Autodesk Inventor part; units mm, degrees
(part 2 of 2)
  line L376 (6.1518, -23.1931) -> (8.2731, -25.3144) projected
  line L377 (8.2731, -25.3144) -> (6.1518, -27.4357) projected
  line L378 (6.1518, -27.4357) -> (4.0305, -25.3144) projected
  line L379 (4.0305, -25.3144) -> (6.1518, -23.1931) projected
  line L380 (3.7123, -25.6326) -> (5.8336, -27.7539) projected
  line L381 (5.8336, -27.7539) -> (3.7123, -29.8753) projected
  line L382 (3.7123, -29.8753) -> (1.591, -27.7539) projected
  line L383 (1.591, -27.7539) -> (3.7123, -25.6326) projected
  line L384 (1.2728, -28.0721) -> (3.3941, -30.1935) projected
  line L385 (3.3941, -30.1935) -> (1.2728, -32.3148) projected
  line L386 (1.2728, -32.3148) -> (-0.8485, -30.1935) projected
  line L387 (-0.8485, -30.1935) -> (1.2728, -28.0721) projected
  line L388 (-1.1667, -30.5117) -> (0.9546, -32.633) projected
  line L389 (0.9546, -32.633) -> (-1.1667, -34.7543) projected
  line L390 (-1.1667, -34.7543) -> (-3.288, -32.633) projected
  line L391 (-3.288, -32.633) -> (-1.1667, -30.5117) projected
  line L392 (-3.6062, -32.9512) -> (-1.4849, -35.0725) projected
  line L393 (-1.4849, -35.0725) -> (-3.6062, -37.1938) projected
  line L394 (-3.6062, -37.1938) -> (-5.7276, -35.0725) projected
  line L395 (-5.7276, -35.0725) -> (-3.6062, -32.9512) projected
  line L396 (-6.0458, -35.3907) -> (-3.9244, -37.512) projected
  line L397 (-3.9244, -37.512) -> (-6.0458, -39.6333) projected
  line L398 (-6.0458, -39.6333) -> (-8.1671, -37.512) projected
  line L399 (-8.1671, -37.512) -> (-6.0458, -35.3907) projected
  line L400 (-8.4853, -37.8302) -> (-6.364, -39.9515) projected
  line L401 (-6.364, -39.9515) -> (-8.4853, -42.0729) projected
  line L402 (-8.4853, -42.0729) -> (-10.6066, -39.9515) projected
  line L403 (-10.6066, -39.9515) -> (-8.4853, -37.8302) projected
  line L404 (28.1075, -6.1165) -> (30.2288, -8.2378) projected
  line L405 (30.2288, -8.2378) -> (28.1075, -10.3591) projected
  line L406 (28.1075, -10.3591) -> (25.9862, -8.2378) projected
  line L407 (25.9862, -8.2378) -> (28.1075, -6.1165) projected
  line L408 (25.668, -8.556) -> (27.7893, -10.6773) projected
  line L409 (27.7893, -10.6773) -> (25.668, -12.7986) projected
  line L410 (25.668, -12.7986) -> (23.5467, -10.6773) projected
  line L411 (23.5467, -10.6773) -> (25.668, -8.556) projected
  line L412 (23.2285, -10.9955) -> (25.3498, -13.1168) projected
  line L413 (25.3498, -13.1168) -> (23.2285, -15.2382) projected
  line L414 (23.2285, -15.2382) -> (21.1071, -13.1168) projected
  line L415 (21.1071, -13.1168) -> (23.2285, -10.9955) projected
  line L416 (20.7889, -13.435) -> (22.9103, -15.5563) projected
  line L417 (22.9103, -15.5563) -> (20.7889, -17.6777) projected
  line L418 (20.7889, -17.6777) -> (18.6676, -15.5563) projected
  line L419 (18.6676, -15.5563) -> (20.7889, -13.435) projected
  line L420 (18.3494, -15.8745) -> (20.4707, -17.9959) projected
  line L421 (20.4707, -17.9959) -> (18.3494, -20.1172) projected
  line L422 (18.3494, -20.1172) -> (16.2281, -17.9959) projected
  line L423 (16.2281, -17.9959) -> (18.3494, -15.8745) projected
  line L424 (15.9099, -18.3141) -> (18.0312, -20.4354) projected
  line L425 (18.0312, -20.4354) -> (15.9099, -22.5567) projected
  line L426 (15.9099, -22.5567) -> (13.7886, -20.4354) projected
  line L427 (13.7886, -20.4354) -> (15.9099, -18.3141) projected
  line L428 (13.4704, -20.7536) -> (15.5917, -22.8749) projected
  line L429 (15.5917, -22.8749) -> (13.4704, -24.9962) projected
  line L430 (13.4704, -24.9962) -> (11.3491, -22.8749) projected
  line L431 (11.3491, -22.8749) -> (13.4704, -20.7536) projected
  line L432 (11.0309, -23.1931) -> (13.1522, -25.3144) projected
  line L433 (13.1522, -25.3144) -> (11.0309, -27.4357) projected
  line L434 (11.0309, -27.4357) -> (8.9095, -25.3144) projected
  line L435 (8.9095, -25.3144) -> (11.0309, -23.1931) projected
  line L436 (8.5913, -25.6326) -> (10.7127, -27.7539) projected
  line L437 (10.7127, -27.7539) -> (8.5913, -29.8753) projected
  line L438 (8.5913, -29.8753) -> (6.47, -27.7539) projected
  line L439 (6.47, -27.7539) -> (8.5913, -25.6326) projected
  line L440 (6.1518, -28.0721) -> (8.2731, -30.1935) projected
  line L441 (8.2731, -30.1935) -> (6.1518, -32.3148) projected
  line L442 (6.1518, -32.3148) -> (4.0305, -30.1935) projected
  line L443 (4.0305, -30.1935) -> (6.1518, -28.0721) projected
  line L444 (3.7123, -30.5117) -> (5.8336, -32.633) projected
  line L445 (5.8336, -32.633) -> (3.7123, -34.7543) projected
  line L446 (3.7123, -34.7543) -> (1.591, -32.633) projected
  line L447 (1.591, -32.633) -> (3.7123, -30.5117) projected
  line L448 (1.2728, -32.9512) -> (3.3941, -35.0725) projected
  line L449 (3.3941, -35.0725) -> (1.2728, -37.1938) projected
  line L450 (1.2728, -37.1938) -> (-0.8485, -35.0725) projected
  line L451 (-0.8485, -35.0725) -> (1.2728, -32.9512) projected
  line L452 (-1.1667, -35.3907) -> (0.9546, -37.512) projected
  line L453 (0.9546, -37.512) -> (-1.1667, -39.6333) projected
  line L454 (-1.1667, -39.6333) -> (-3.288, -37.512) projected
  line L455 (-3.288, -37.512) -> (-1.1667, -35.3907) projected
  line L456 (-3.6062, -37.8302) -> (-1.4849, -39.9515) projected
  line L457 (-1.4849, -39.9515) -> (-3.6062, -42.0729) projected
  line L458 (-3.6062, -42.0729) -> (-5.7276, -39.9515) projected
  line L459 (-5.7276, -39.9515) -> (-3.6062, -37.8302) projected
  line L460 (30.547, -8.556) -> (32.6683, -10.6773) projected
  line L461 (32.6683, -10.6773) -> (30.547, -12.7986) projected
  line L462 (30.547, -12.7986) -> (28.4257, -10.6773) projected
  line L463 (28.4257, -10.6773) -> (30.547, -8.556) projected
  line L464 (28.1075, -10.9955) -> (30.2288, -13.1168) projected
  line L465 (30.2288, -13.1168) -> (28.1075, -15.2382) projected
  line L466 (28.1075, -15.2382) -> (25.9862, -13.1168) projected
  line L467 (25.9862, -13.1168) -> (28.1075, -10.9955) projected
  line L468 (25.668, -13.435) -> (27.7893, -15.5563) projected
  line L469 (27.7893, -15.5563) -> (25.668, -17.6777) projected
  line L470 (25.668, -17.6777) -> (23.5467, -15.5563) projected
  line L471 (23.5467, -15.5563) -> (25.668, -13.435) projected
  line L472 (23.2285, -15.8745) -> (25.3498, -17.9959) projected
  line L473 (25.3498, -17.9959) -> (23.2285, -20.1172) projected
  line L474 (23.2285, -20.1172) -> (21.1071, -17.9959) projected
  line L475 (21.1071, -17.9959) -> (23.2285, -15.8745) projected
  line L476 (15.9099, -23.1931) -> (18.0312, -25.3144) projected
  line L477 (18.0312, -25.3144) -> (15.9099, -27.4357) projected
  line L478 (15.9099, -27.4357) -> (13.7886, -25.3144) projected
  line L479 (13.7886, -25.3144) -> (15.9099, -23.1931) projected
  line L480 (13.4704, -25.6326) -> (15.5917, -27.7539) projected
  line L481 (15.5917, -27.7539) -> (13.4704, -29.8753) projected
  line L482 (13.4704, -29.8753) -> (11.3491, -27.7539) projected
  line L483 (11.3491, -27.7539) -> (13.4704, -25.6326) projected
  line L484 (11.0309, -28.0721) -> (13.1522, -30.1935) projected
  line L485 (13.1522, -30.1935) -> (11.0309, -32.3148) projected
  line L486 (11.0309, -32.3148) -> (8.9095, -30.1935) projected
  line L487 (8.9095, -30.1935) -> (11.0309, -28.0721) projected
  line L488 (8.5913, -30.5117) -> (10.7127, -32.633) projected
  line L489 (10.7127, -32.633) -> (8.5913, -34.7543) projected
  line L490 (8.5913, -34.7543) -> (6.47, -32.633) projected
  line L491 (6.47, -32.633) -> (8.5913, -30.5117) projected
  line L492 (6.1518, -32.9512) -> (8.2731, -35.0725) projected
  line L493 (8.2731, -35.0725) -> (6.1518, -37.1938) projected
  line L494 (6.1518, -37.1938) -> (4.0305, -35.0725) projected
  line L495 (4.0305, -35.0725) -> (6.1518, -32.9512) projected
  line L496 (3.7123, -35.3907) -> (5.8336, -37.512) projected
  line L497 (5.8336, -37.512) -> (3.7123, -39.6333) projected
  line L498 (3.7123, -39.6333) -> (1.591, -37.512) projected
  line L499 (1.591, -37.512) -> (3.7123, -35.3907) projected
  line L500 (1.2728, -37.8302) -> (3.3941, -39.9515) projected
  line L501 (3.3941, -39.9515) -> (1.2728, -42.0729) projected
  line L502 (1.2728, -42.0729) -> (-0.8485, -39.9515) projected
  line L503 (-0.8485, -39.9515) -> (1.2728, -37.8302) projected
  line L504 (32.9865, -10.9955) -> (35.1079, -13.1168) projected
  line L505 (35.1079, -13.1168) -> (32.9865, -15.2382) projected
  line L506 (32.9865, -15.2382) -> (30.8652, -13.1168) projected
  line L507 (30.8652, -13.1168) -> (32.9865, -10.9955) projected
  line L508 (13.4704, -30.5117) -> (15.5917, -32.633) projected
  line L509 (15.5917, -32.633) -> (13.4704, -34.7543) projected
  line L510 (13.4704, -34.7543) -> (11.3491, -32.633) projected
  line L511 (11.3491, -32.633) -> (13.4704, -30.5117) projected
  line L512 (11.0309, -32.9512) -> (13.1522, -35.0725) projected
  line L513 (13.1522, -35.0725) -> (11.0309, -37.1938) projected
  line L514 (11.0309, -37.1938) -> (8.9095, -35.0725) projected
  line L515 (8.9095, -35.0725) -> (11.0309, -32.9512) projected
  line L516 (8.5913, -35.3907) -> (10.7127, -37.512) projected
  line L517 (10.7127, -37.512) -> (8.5913, -39.6333) projected
  line L518 (8.5913, -39.6333) -> (6.47, -37.512) projected
  line L519 (6.47, -37.512) -> (8.5913, -35.3907) projected
  line L520 (6.1518, -37.8302) -> (8.2731, -39.9515) projected
  line L521 (8.2731, -39.9515) -> (6.1518, -42.0729) projected
  line L522 (6.1518, -42.0729) -> (4.0305, -39.9515) projected
  line L523 (4.0305, -39.9515) -> (6.1518, -37.8302) projected
  line L524 (35.426, -13.435) -> (37.5474, -15.5563) projected
  line L525 (37.5474, -15.5563) -> (35.426, -17.6777) projected
  line L526 (35.426, -17.6777) -> (33.3047, -15.5563) projected
  line L527 (33.3047, -15.5563) -> (35.426, -13.435) projected
  line L528 (28.1075, -20.7536) -> (30.2288, -22.8749) projected
  line L529 (30.2288, -22.8749) -> (28.1075, -24.9962) projected
  line L530 (28.1075, -24.9962) -> (25.9862, -22.8749) projected
  line L531 (25.9862, -22.8749) -> (28.1075, -20.7536) projected
  line L532 (25.668, -23.1931) -> (27.7893, -25.3144) projected
  line L533 (27.7893, -25.3144) -> (25.668, -27.4357) projected
  line L534 (25.668, -27.4357) -> (23.5467, -25.3144) projected
  line L535 (23.5467, -25.3144) -> (25.668, -23.1931) projected
  line L536 (23.2285, -25.6326) -> (25.3498, -27.7539) projected
  line L537 (25.3498, -27.7539) -> (23.2285, -29.8753) projected
  line L538 (23.2285, -29.8753) -> (21.1071, -27.7539) projected
  line L539 (21.1071, -27.7539) -> (23.2285, -25.6326) projected
  line L540 (18.3494, -30.5117) -> (20.4707, -32.633) projected
  line L541 (20.4707, -32.633) -> (18.3494, -34.7543) projected
  line L542 (18.3494, -34.7543) -> (16.2281, -32.633) projected
  line L543 (16.2281, -32.633) -> (18.3494, -30.5117) projected
  line L544 (15.9099, -32.9512) -> (18.0312, -35.0725) projected
  line L545 (18.0312, -35.0725) -> (15.9099, -37.1938) projected
  line L546 (15.9099, -37.1938) -> (13.7886, -35.0725) projected
  line L547 (13.7886, -35.0725) -> (15.9099, -32.9512) projected
  line L548 (13.4704, -35.3907) -> (15.5917, -37.512) projected
  line L549 (15.5917, -37.512) -> (13.4704, -39.6333) projected
  line L550 (13.4704, -39.6333) -> (11.3491, -37.512) projected
  line L551 (11.3491, -37.512) -> (13.4704, -35.3907) projected
  line L552 (11.0309, -37.8302) -> (13.1522, -39.9515) projected
  line L553 (13.1522, -39.9515) -> (11.0309, -42.0729) projected
  line L554 (11.0309, -42.0729) -> (8.9095, -39.9515) projected
  line L555 (8.9095, -39.9515) -> (11.0309, -37.8302) projected
  line L556 (8.5913, -40.2697) -> (10.7127, -42.3911) projected
  line L557 (10.7127, -42.3911) -> (8.5913, -44.5124) projected
  line L558 (8.5913, -44.5124) -> (6.47, -42.3911) projected
  line L559 (6.47, -42.3911) -> (8.5913, -40.2697) projected
  line L560 (32.9865, -20.7536) -> (35.1079, -22.8749) projected
  line L561 (35.1079, -22.8749) -> (32.9865, -24.9962) projected
  line L562 (32.9865, -24.9962) -> (30.8652, -22.8749) projected
  line L563 (30.8652, -22.8749) -> (32.9865, -20.7536) projected
  line L564 (30.547, -23.1931) -> (32.6683, -25.3144) projected
  line L565 (32.6683, -25.3144) -> (30.547, -27.4357) projected
  line L566 (30.547, -27.4357) -> (28.4257, -25.3144) projected
  line L567 (28.4257, -25.3144) -> (30.547, -23.1931) projected
  line L568 (28.1075, -25.6326) -> (30.2288, -27.7539) projected
  line L569 (30.2288, -27.7539) -> (28.1075, -29.8753) projected
  line L570 (28.1075, -29.8753) -> (25.9862, -27.7539) projected
  line L571 (25.9862, -27.7539) -> (28.1075, -25.6326) projected
  line L572 (25.668, -28.0721) -> (27.7893, -30.1935) projected
  line L573 (27.7893, -30.1935) -> (25.668, -32.3148) projected
  line L574 (25.668, -32.3148) -> (23.5467, -30.1935) projected
  line L575 (23.5467, -30.1935) -> (25.668, -28.0721) projected
  line L576 (23.2285, -30.5117) -> (25.3498, -32.633) projected
  line L577 (25.3498, -32.633) -> (23.2285, -34.7543) projected
  line L578 (23.2285, -34.7543) -> (21.1071, -32.633) projected
  line L579 (21.1071, -32.633) -> (23.2285, -30.5117) projected
  line L580 (20.7889, -32.9512) -> (22.9103, -35.0725) projected
  line L581 (22.9103, -35.0725) -> (20.7889, -37.1938) projected
  line L582 (20.7889, -37.1938) -> (18.6676, -35.0725) projected
  line L583 (18.6676, -35.0725) -> (20.7889, -32.9512) projected
  line L584 (18.3494, -35.3907) -> (20.4707, -37.512) projected
  line L585 (20.4707, -37.512) -> (18.3494, -39.6333) projected
  line L586 (18.3494, -39.6333) -> (16.2281, -37.512) projected
  line L587 (16.2281, -37.512) -> (18.3494, -35.3907) projected
  line L588 (15.9099, -37.8302) -> (18.0312, -39.9515) projected
  line L589 (18.0312, -39.9515) -> (15.9099, -42.0729) projected
  line L590 (15.9099, -42.0729) -> (13.7886, -39.9515) projected
  line L591 (13.7886, -39.9515) -> (15.9099, -37.8302) projected
  line L592 (13.4704, -40.2697) -> (15.5917, -42.3911) projected
  line L593 (15.5917, -42.3911) -> (13.4704, -44.5124) projected
  line L594 (13.4704, -44.5124) -> (11.3491, -42.3911) projected
  line L595 (11.3491, -42.3911) -> (13.4704, -40.2697) projected
  line L596 (37.8656, -20.7536) -> (39.9869, -22.8749) projected
  line L597 (39.9869, -22.8749) -> (37.8656, -24.9962) projected
  line L598 (37.8656, -24.9962) -> (35.7442, -22.8749) projected
  line L599 (35.7442, -22.8749) -> (37.8656, -20.7536) projected
  line L600 (35.426, -23.1931) -> (37.5474, -25.3144) projected
  line L601 (37.5474, -25.3144) -> (35.426, -27.4357) projected
  line L602 (35.426, -27.4357) -> (33.3047, -25.3144) projected
  line L603 (33.3047, -25.3144) -> (35.426, -23.1931) projected
  line L604 (32.9865, -25.6326) -> (35.1079, -27.7539) projected
  line L605 (35.1079, -27.7539) -> (32.9865, -29.8753) projected
  line L606 (32.9865, -29.8753) -> (30.8652, -27.7539) projected
  line L607 (30.8652, -27.7539) -> (32.9865, -25.6326) projected
  line L608 (30.547, -28.0721) -> (32.6683, -30.1935) projected
  line L609 (32.6683, -30.1935) -> (30.547, -32.3148) projected
  line L610 (30.547, -32.3148) -> (28.4257, -30.1935) projected
  line L611 (28.4257, -30.1935) -> (30.547, -28.0721) projected
  line L612 (28.1075, -30.5117) -> (30.2288, -32.633) projected
  line L613 (30.2288, -32.633) -> (28.1075, -34.7543) projected
  line L614 (28.1075, -34.7543) -> (25.9862, -32.633) projected
  line L615 (25.9862, -32.633) -> (28.1075, -30.5117) projected
  line L616 (25.668, -32.9512) -> (27.7893, -35.0725) projected
  line L617 (27.7893, -35.0725) -> (25.668, -37.1938) projected
  line L618 (25.668, -37.1938) -> (23.5467, -35.0725) projected
  line L619 (23.5467, -35.0725) -> (25.668, -32.9512) projected
  line L620 (23.2285, -35.3907) -> (25.3498, -37.512) projected
  line L621 (25.3498, -37.512) -> (23.2285, -39.6333) projected
  line L622 (23.2285, -39.6333) -> (21.1071, -37.512) projected
  line L623 (21.1071, -37.512) -> (23.2285, -35.3907) projected
  line L624 (18.3494, -40.2697) -> (20.4707, -42.3911) projected
  line L625 (20.4707, -42.3911) -> (18.3494, -44.5124) projected
  line L626 (18.3494, -44.5124) -> (16.2281, -42.3911) projected
  line L627 (16.2281, -42.3911) -> (18.3494, -40.2697) projected
  line L628 (37.8656, -25.6326) -> (39.9869, -27.7539) projected
  line L629 (39.9869, -27.7539) -> (37.8656, -29.8753) projected
  line L630 (37.8656, -29.8753) -> (35.7442, -27.7539) projected
  line L631 (35.7442, -27.7539) -> (37.8656, -25.6326) projected
  line L632 (35.426, -28.0721) -> (37.5474, -30.1935) projected
  line L633 (37.5474, -30.1935) -> (35.426, -32.3148) projected
  line L634 (35.426, -32.3148) -> (33.3047, -30.1935) projected
  line L635 (33.3047, -30.1935) -> (35.426, -28.0721) projected
  line L636 (32.9865, -30.5117) -> (35.1079, -32.633) projected
  line L637 (35.1079, -32.633) -> (32.9865, -34.7543) projected
  line L638 (32.9865, -34.7543) -> (30.8652, -32.633) projected
  line L639 (30.8652, -32.633) -> (32.9865, -30.5117) projected
  line L640 (30.547, -32.9512) -> (32.6683, -35.0725) projected
  line L641 (32.6683, -35.0725) -> (30.547, -37.1938) projected
  line L642 (30.547, -37.1938) -> (28.4257, -35.0725) projected
  line L643 (28.4257, -35.0725) -> (30.547, -32.9512) projected
  line L644 (28.1075, -35.3907) -> (30.2288, -37.512) projected
  line L645 (30.2288, -37.512) -> (28.1075, -39.6333) projected
  line L646 (28.1075, -39.6333) -> (25.9862, -37.512) projected
  line L647 (25.9862, -37.512) -> (28.1075, -35.3907) projected
  line L648 (25.668, -37.8302) -> (27.7893, -39.9515) projected
  line L649 (27.7893, -39.9515) -> (25.668, -42.0729) projected
  line L650 (25.668, -42.0729) -> (23.5467, -39.9515) projected
  line L651 (23.5467, -39.9515) -> (25.668, -37.8302) projected
  line L652 (40.3051, -28.0721) -> (42.4264, -30.1935) projected
  line L653 (42.4264, -30.1935) -> (40.3051, -32.3148) projected
  line L654 (40.3051, -32.3148) -> (38.1838, -30.1935) projected
  line L655 (38.1838, -30.1935) -> (40.3051, -28.0721) projected
  line L656 (37.8656, -30.5117) -> (39.9869, -32.633) projected
  line L657 (39.9869, -32.633) -> (37.8656, -34.7543) projected
  line L658 (37.8656, -34.7543) -> (35.7442, -32.633) projected
  line L659 (35.7442, -32.633) -> (37.8656, -30.5117) projected
  line L660 (35.426, -32.9512) -> (37.5474, -35.0725) projected
  line L661 (37.5474, -35.0725) -> (35.426, -37.1938) projected
  line L662 (35.426, -37.1938) -> (33.3047, -35.0725) projected
  line L663 (33.3047, -35.0725) -> (35.426, -32.9512) projected
  line L664 (32.9865, -35.3907) -> (35.1079, -37.512) projected
  line L665 (35.1079, -37.512) -> (32.9865, -39.6333) projected
  line L666 (32.9865, -39.6333) -> (30.8652, -37.512) projected
  line L667 (30.8652, -37.512) -> (32.9865, -35.3907) projected
  line L668 (30.547, -37.8302) -> (32.6683, -39.9515) projected
  line L669 (32.6683, -39.9515) -> (30.547, -42.0729) projected
  line L670 (30.547, -42.0729) -> (28.4257, -39.9515) projected
  line L671 (28.4257, -39.9515) -> (30.547, -37.8302) projected
  line L672 (40.3051, -32.9512) -> (42.4264, -35.0725) projected
  line L673 (42.4264, -35.0725) -> (40.3051, -37.1938) projected
  line L674 (40.3051, -37.1938) -> (38.1838, -35.0725) projected
  line L675 (38.1838, -35.0725) -> (40.3051, -32.9512) projected
  line L676 (37.8656, -35.3907) -> (39.9869, -37.512) projected
  line L677 (39.9869, -37.512) -> (37.8656, -39.6333) projected
  line L678 (37.8656, -39.6333) -> (35.7442, -37.512) projected
  line L679 (35.7442, -37.512) -> (37.8656, -35.3907) projected
  line L680 (35.426, -37.8302) -> (37.5474, -39.9515) projected
  line L681 (37.5474, -39.9515) -> (35.426, -42.0729) projected
  line L682 (35.426, -42.0729) -> (33.3047, -39.9515) projected
  line L683 (33.3047, -39.9515) -> (35.426, -37.8302) projected
  line L684 (29.4532, -43.8031) -> (30.547, -42.7092) projected
  line L685 (30.547, -42.7092) -> (31.7996, -43.9618) projected
  arc A0 (31.7996, -43.9618) -> (32.4051, -43.9309) centre (31.4663, -31.4663) ccw projected
  line L686 (32.4051, -43.9309) -> (30.8652, -42.3911) projected
  line L687 (30.8652, -42.3911) -> (32.9865, -40.2697) projected
  line L688 (32.9865, -40.2697) -> (35.1079, -42.3911) projected
  line L689 (35.1079, -42.3911) -> (33.7415, -43.7574) projected
  arc A1 (33.7415, -43.7574) -> (43.7574, -33.7415) centre (31.4663, -31.4663) ccw projected
  line L690 (43.7574, -33.7415) -> (42.7446, -34.7543) projected
  line L691 (42.7446, -34.7543) -> (40.6233, -32.633) projected
  line L692 (40.6233, -32.633) -> (42.7446, -30.5117) projected
  line L693 (42.7446, -30.5117) -> (43.9635, -31.7305) projected
  arc A2 (43.9635, -31.7305) -> (43.9606, -31.0913) centre (31.4663, -31.4663) ccw projected
  line L694 (43.9606, -31.0913) -> (43.0628, -30.1935) projected
  line L695 (43.0628, -30.1935) -> (43.8031, -29.4532) projected
  arc A3 (43.8031, -29.4532) -> (43.7034, -28.9164) centre (31.4663, -31.4663) ccw projected
  line L696 (43.7034, -28.9164) -> (42.7446, -29.8753) projected
  line L697 (42.7446, -29.8753) -> (40.6233, -27.7539) projected
  line L698 (40.6233, -27.7539) -> (42.5978, -25.7795) projected
  arc A4 (42.5978, -25.7795) -> (42.376, -25.3648) centre (31.4663, -31.4663) ccw projected
  line L699 (42.376, -25.3648) -> (40.3051, -27.4357) projected
  line L700 (40.3051, -27.4357) -> (38.1838, -25.3144) projected
  line L701 (38.1838, -25.3144) -> (40.3051, -23.1931) projected
  line L702 (40.3051, -23.1931) -> (42.2404, -25.1284) projected
  arc A5 (42.2404, -25.1284) -> (37.4767, -20.5061) centre (31.4663, -31.4663) ccw projected
  line L703 (37.4767, -20.5061) -> (35.426, -22.5567) projected
  line L704 (35.426, -22.5567) -> (33.3047, -20.4354) projected
  line L705 (33.3047, -20.4354) -> (34.4199, -19.3202) projected
  arc A6 (34.4199, -19.3202) -> (33.8985, -19.2052) centre (31.4663, -31.4663) ccw projected
  line L706 (33.8985, -19.2052) -> (32.9865, -20.1172) projected
  line L707 (32.9865, -20.1172) -> (31.8412, -18.9719) projected
  arc A7 (31.8412, -18.9719) -> (31.202, -18.969) centre (31.4663, -31.4663) ccw projected
  line L708 (31.202, -18.969) -> (32.6683, -20.4354) projected
  line L709 (32.6683, -20.4354) -> (30.547, -22.5567) projected
  line L710 (30.547, -22.5567) -> (28.4257, -20.4354) projected
  line L711 (28.4257, -20.4354) -> (29.7807, -19.0804) projected
  arc A8 (29.7807, -19.0804) -> (29.0159, -19.2088) centre (31.4663, -31.4663) ccw projected
  line L712 (29.0159, -19.2088) -> (28.1075, -20.1172) projected
  line L713 (28.1075, -20.1172) -> (27.577, -19.5867) projected
  arc A9 (27.577, -19.5867) -> (27.1055, -19.7516) centre (31.4663, -31.4663) ccw projected
  line L714 (27.1055, -19.7516) -> (27.7893, -20.4354) projected
  line L715 (27.7893, -20.4354) -> (25.668, -22.5567) projected
  line L716 (25.668, -22.5567) -> (24.321, -21.2098) projected
  arc A10 (24.321, -21.2098) -> (23.9519, -21.477) centre (31.4663, -31.4663) ccw projected
  line L717 (23.9519, -21.477) -> (25.3498, -22.8749) projected
  line L718 (25.3498, -22.8749) -> (23.2285, -24.9962) projected
  line L719 (23.2285, -24.9962) -> (21.7878, -23.5556) projected
  arc A11 (21.7878, -23.5556) -> (21.5075, -23.9116) centre (31.4663, -31.4663) ccw projected
  line L720 (21.5075, -23.9116) -> (22.9103, -25.3144) projected
  line L721 (22.9103, -25.3144) -> (20.7889, -27.4357) projected
  line L722 (20.7889, -27.4357) -> (19.9526, -26.5994) projected
  arc A12 (19.9526, -26.5994) -> (19.7708, -27.054) centre (31.4663, -31.4663) ccw projected
  line L723 (19.7708, -27.054) -> (20.4707, -27.7539) projected
  line L724 (20.4707, -27.7539) -> (19.2088, -29.0159) projected
  arc A13 (19.2088, -29.0159) -> (19.0804, -29.7807) centre (31.4663, -31.4663) ccw projected
  line L725 (19.0804, -29.7807) -> (20.7889, -28.0721) projected
  line L726 (20.7889, -28.0721) -> (22.9103, -30.1935) projected
  line L727 (22.9103, -30.1935) -> (20.7889, -32.3148) projected
  line L728 (20.7889, -32.3148) -> (18.6676, -30.1935) projected
  line L729 (18.6676, -30.1935) -> (18.914, -29.9471) projected
  line L730 (18.0124, -30.2123) -> (18.914, -29.9471) projected
  line L731 (18.0124, -30.2123) -> (15.9099, -32.3148) projected
  line L732 (15.9099, -32.3148) -> (13.7886, -30.1935) projected
  line L733 (13.7886, -30.1935) -> (15.9099, -28.0721) projected
  line L734 (15.9099, -28.0721) -> (17.5736, -29.7358) projected
  arc A14 (17.6542, -29.18) -> (17.5736, -29.7358) centre (31.4663, -31.4663) ccw projected
  line L735 (17.6542, -29.18) -> (16.2281, -27.7539) projected
  line L736 (16.2281, -27.7539) -> (18.3494, -25.6326) projected
  line L737 (18.3494, -25.6326) -> (18.6193, -25.9025) projected
  arc A15 (18.8179, -25.4647) -> (18.6193, -25.9025) centre (31.4663, -31.4663) ccw projected
  line L738 (18.8179, -25.4647) -> (18.6676, -25.3144) projected
  line L739 (18.6676, -25.3144) -> (19.124, -24.8581) projected
  arc A16 (20.2276, -23.1181) -> (19.124, -24.8581) centre (31.4663, -31.4663) ccw projected
  line L740 (20.2276, -23.1181) -> (18.3494, -24.9962) projected
  line L741 (18.3494, -24.9962) -> (16.2281, -22.8749) projected
  line L742 (16.2281, -22.8749) -> (18.3494, -20.7536) projected
  line L743 (18.3494, -20.7536) -> (20.4379, -22.8421) projected
  arc A17 (20.7224, -22.4902) -> (20.4379, -22.8421) centre (31.4663, -31.4663) ccw projected
  line L744 (20.7224, -22.4902) -> (18.6676, -20.4354) projected
  line L745 (18.6676, -20.4354) -> (20.7889, -18.3141) projected
  line L746 (20.7889, -18.3141) -> (22.8818, -20.407) projected
  arc A18 (24.8581, -19.124) -> (22.8818, -20.407) centre (31.4663, -31.4663) ccw projected
  line L747 (24.8581, -19.124) -> (25.668, -18.3141) projected
  line L748 (25.668, -18.3141) -> (25.9519, -18.598) projected
  arc A19 (26.4039, -18.4136) -> (25.9519, -18.598) centre (31.4663, -31.4663) ccw projected
  line L749 (26.4039, -18.4136) -> (25.9862, -17.9959) projected
  line L750 (25.9862, -17.9959) -> (28.1075, -15.8745) projected
  line L751 (28.1075, -15.8745) -> (29.7988, -17.5659) projected
  arc A20 (30.378, -17.5086) -> (29.7988, -17.5659) centre (31.4663, -31.4663) ccw projected
  line L752 (30.378, -17.5086) -> (28.4257, -15.5563) projected
  line L753 (28.4257, -15.5563) -> (30.547, -13.435) projected
  line L754 (30.547, -13.435) -> (32.6683, -15.5563) projected
  line L755 (32.6683, -15.5563) -> (30.7396, -17.4851) projected
  arc A21 (31.3946, -17.4664) -> (30.7396, -17.4851) centre (31.4663, -31.4663) ccw projected
  line L756 (31.3946, -17.4664) -> (32.9865, -15.8745) projected
  line L757 (32.9865, -15.8745) -> (35.0428, -17.9308) projected
  arc A22 (35.9531, -18.2047) -> (35.0428, -17.9308) centre (31.4663, -31.4663) ccw projected
  line L758 (35.9531, -18.2047) -> (35.7442, -17.9959) projected
  line L759 (35.7442, -17.9959) -> (37.8656, -15.8745) projected
  line L760 (37.8656, -15.8745) -> (39.248, -17.257) projected
  line L761 (39.248, -17.257) -> (38.2823, -15.6549) projected
  line L762 (38.2823, -15.6549) -> (38.1838, -15.5563) projected
  line L763 (38.1838, -15.5563) -> (38.2082, -15.5319) projected
  line L764 (38.2082, -15.5319) -> (37.9689, -15.1349) projected
  line L765 (37.9689, -15.1349) -> (37.8656, -15.2382) projected
  line L766 (37.8656, -15.2382) -> (35.7442, -13.1168) projected
  line L767 (35.7442, -13.1168) -> (36.3733, -12.4878) projected
  line L768 (36.3733, -12.4878) -> (36.1339, -12.0907) projected
  line L769 (36.1339, -12.0907) -> (35.426, -12.7986) projected
  line L770 (35.426, -12.7986) -> (33.3047, -10.6773) projected
  line L771 (33.3047, -10.6773) -> (34.5384, -9.4437) projected
  line L772 (34.5384, -9.4437) -> (34.299, -9.0466) projected
  line L773 (34.299, -9.0466) -> (32.9865, -10.3591) projected
  line L774 (32.9865, -10.3591) -> (30.8652, -8.2378) projected
  line L775 (30.8652, -8.2378) -> (32.7035, -6.3995) projected
  line L776 (32.7035, -6.3995) -> (32.4641, -6.0025) projected
  line L777 (32.4641, -6.0025) -> (30.547, -7.9196) projected
  line L778 (30.547, -7.9196) -> (28.4257, -5.7983) projected
  line L779 (28.4257, -5.7983) -> (30.547, -3.677) projected
  line L780 (30.547, -3.677) -> (31.8444, -4.9744) projected
  line L781 (31.8444, -4.9744) -> (29.6985, -1.4142) projected
  line L782 (29.6985, -1.4142) -> (15.9099, 12.3744) projected
  line L783 (15.9099, 12.3744) -> (-26.5165, -30.052) projected
  line L784 (-26.5165, -30.052) -> (-12.7279, -43.8406) projected
  line L785 (-12.7279, -43.8406) -> (-11.5531, -43.8841) projected
  line L786 (-11.5531, -43.8841) -> (-13.0461, -42.3911) projected
  line L787 (-13.0461, -42.3911) -> (-10.9248, -40.2697) projected
  line L788 (-10.9248, -40.2697) -> (-8.8035, -42.3911) projected
  line L789 (-8.8035, -42.3911) -> (-10.3414, -43.9289) projected
  line L790 (-10.3414, -43.9289) -> (-9.7277, -43.9516) projected
  line L791 (-9.7277, -43.9516) -> (-8.4853, -42.7092) projected
  line L792 (-8.4853, -42.7092) -> (-7.1474, -44.0471) projected
  line L793 (-7.1474, -44.0471) -> (-6.4866, -44.0716) projected
  line L794 (-6.4866, -44.0716) -> (-8.1671, -42.3911) projected
  line L795 (-8.1671, -42.3911) -> (-6.0458, -40.2697) projected
  line L796 (-6.0458, -40.2697) -> (-3.9244, -42.3911) projected
  line L797 (-3.9244, -42.3911) -> (-5.6364, -44.103) projected
  line L798 (-5.6364, -44.103) -> (-5.0227, -44.1257) projected
  line L799 (-5.0227, -44.1257) -> (-3.6062, -42.7092) projected
  line L800 (-3.6062, -42.7092) -> (-2.0809, -44.2346) projected
  line L801 (-2.0809, -44.2346) -> (-1.4201, -44.259) projected
  line L802 (-1.4201, -44.259) -> (-3.288, -42.3911) projected
  line L803 (-3.288, -42.3911) -> (-1.1667, -40.2697) projected
  line L804 (-1.1667, -40.2697) -> (0.9546, -42.3911) projected
  line L805 (0.9546, -42.3911) -> (-0.9315, -44.2771) projected
  line L806 (-0.9315, -44.2771) -> (-0.3178, -44.2998) projected
  line L807 (-0.3178, -44.2998) -> (1.2728, -42.7092) projected
  line L808 (1.2728, -42.7092) -> (2.9856, -44.422) projected
  line L809 (2.9856, -44.422) -> (3.6464, -44.4465) projected
  line L810 (3.6464, -44.4465) -> (1.591, -42.3911) projected
  line L811 (1.591, -42.3911) -> (3.7123, -40.2697) projected
  line L812 (3.7123, -40.2697) -> (5.8336, -42.3911) projected
  line L813 (5.8336, -42.3911) -> (3.7735, -44.4512) projected
  line L814 (3.7735, -44.4512) -> (4.3872, -44.4739) projected
  line L815 (4.3872, -44.4739) -> (6.1518, -42.7092) projected
  line L816 (6.1518, -42.7092) -> (8.0521, -44.6095) projected
  line L817 (8.0521, -44.6095) -> (9.0921, -44.648) projected
  line L818 (9.0921, -44.648) -> (11.0309, -42.7092) projected
  line L819 (11.0309, -42.7092) -> (13.1186, -44.797) projected
  line L820 (13.1186, -44.797) -> (13.7971, -44.8221) projected
  line L821 (13.7971, -44.8221) -> (15.9099, -42.7092) projected
  line L822 (15.9099, -42.7092) -> (18.0312, -44.8306) projected
  line L823 (18.0312, -44.8306) -> (17.8884, -44.9734) projected
  line L824 (17.8884, -44.9734) -> (18.8459, -45.0089) projected
  line L825 (18.8459, -45.0089) -> (18.6676, -44.8306) projected
  line L826 (18.6676, -44.8306) -> (20.7889, -42.7092) projected
  line L827 (20.7889, -42.7092) -> (22.9103, -44.8306) projected
  line L828 (22.9103, -44.8306) -> (22.5933, -45.1475) projected
  line L829 (22.5933, -45.1475) -> (23.207, -45.1702) projected
  line L830 (23.207, -45.1702) -> (23.2285, -45.1488) projected
  line L831 (23.2285, -45.1488) -> (23.2516, -45.1719) projected
  line L832 (23.2516, -45.1719) -> (23.9124, -45.1963) projected
  line L833 (23.9124, -45.1963) -> (23.5467, -44.8306) projected
  line L834 (23.5467, -44.8306) -> (24.6708, -43.7064) projected
  arc A23 (24.2673, -43.4735) -> (24.6708, -43.7064) centre (31.4663, -31.4663) ccw projected
  line L835 (24.2673, -43.4735) -> (23.2285, -44.5124) projected
  line L836 (23.2285, -44.5124) -> (21.1071, -42.3911) projected
  line L837 (21.1071, -42.3911) -> (21.8536, -41.6445) projected
  arc A24 (21.5315, -41.3303) -> (21.8536, -41.6445) centre (31.4663, -31.4663) ccw projected
  line L838 (21.5315, -41.3303) -> (20.7889, -42.0729) projected
  line L839 (20.7889, -42.0729) -> (18.6676, -39.9515) projected
  line L840 (18.6676, -39.9515) -> (20.7889, -37.8302) projected
  line L841 (20.7889, -37.8302) -> (22.9103, -39.9515) projected
  line L842 (22.9103, -39.9515) -> (22.5921, -40.2697) projected
  arc A25 (22.5921, -40.2697) -> (22.9148, -40.5834) centre (31.4663, -31.4663) ccw projected
  line L843 (22.9148, -40.5834) -> (23.2285, -40.2697) projected
  line L844 (23.2285, -40.2697) -> (25.2959, -42.3372) projected
  arc A26 (25.2959, -42.3372) -> (26.557, -42.9619) centre (31.4663, -31.4663) ccw projected
  line L845 (26.557, -42.9619) -> (25.9862, -42.3911) projected
  line L846 (25.9862, -42.3911) -> (28.1075, -40.2697) projected
  line L847 (28.1075, -40.2697) -> (30.2288, -42.3911) projected
  line L848 (30.2288, -42.3911) -> (28.9164, -43.7034) projected
  arc A27 (28.9164, -43.7034) -> (29.4532, -43.8031) centre (31.4663, -31.4663) ccw projected
  line L849 (-43.8969, -11.5402) -> (-45.3549, 28)
  point P0 (0, 0)
  constraints: 2 end point
sketch "Sketch19" plane through (-54.5, 0, 54.5) normal (0.7071068, 0, 0.7071068) x (0.7071068, 0, -0.7071068)
  line L0 (64, 7) -> (89.5339, 7)
  line L1 (89.5339, 7) -> (89.5339, 0.7391)
  line L2 (89.5339, 0.7391) -> (64, 0.7391)
  line L3 (64, 0.7391) -> (64, 7)
  line L4 (65.4876, 7) -> (65.4876, 0.7391)
  line L5 (64, 5.5484) -> (89.5339, 5.5484)
  line L6 (68.4876, 7) -> (68.4876, 0.7391)
  line L7 (71.4876, 7) -> (71.4876, 0.7391)
  line L8 (74.4876, 7) -> (74.4876, 0.7391)
  line L9 (77.4876, 7) -> (77.4876, 0.7391)
  line L10 (80.4876, 7) -> (80.4876, 0.7391)
  line L11 (83.4876, 7) -> (83.4876, 0.7391)
  line L12 (86.4876, 7) -> (86.4876, 0.7391)
  line L13 (89.4876, 7) -> (89.4876, 0.7391)
  line L14 (64, 3.5484) -> (89.5339, 3.5484)
  line L15 (64, 1.5484) -> (89.5339, 1.5484)
  point P0 (77.0746, 0)
  dimension "d95" = 3
  dimension "d102" = 2
  constraints: 32 end point, 4 point on line, 3 perpendicular, 2 horizontal, 1 parallel, 1 vertical, 30 other
  measures "d95" distance of L4.start L6.start
  measures "d102" distance of L5.start L14.start
body "Solid1"
